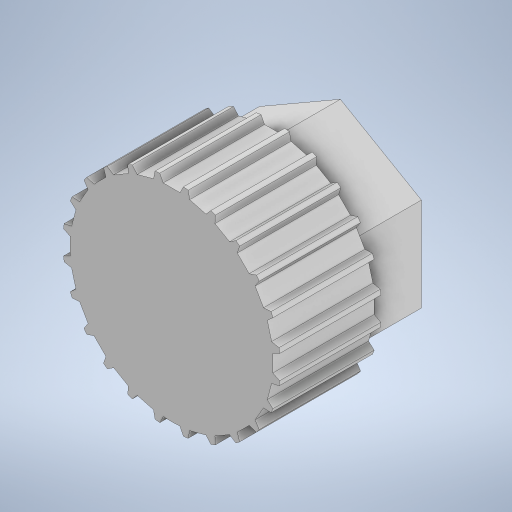
# Autodesk Inventor part: Nastavek Maillard Freewheel Tool
Saved by Autodesk Inventor 2023.3 (Build 273359000, 359)
## iProperties
Created: 2024-05-29
Part Number: Nastavek Maillard Freewheel Tool
Material: Generic
Document SubType Name: Modeling
Designer: David Zindović
Density: 1 g/cm^3
Appearance: Default
Author: David Zindović
Autodesk Inventor part; units mm, degrees
ref_plane "YZ Plane" through (0, 0, 0) normal (1, 0, 0) x (0, 1, 0)
ref_plane "XZ Plane" through (0, 0, 0) normal (0, 1, 0) x (-1, 0, 0)
ref_plane "XY Plane" through (0, 0, 0) normal (0, 0, 1) x (1, 0, 0)
sketch "Sketch1" plane through (0, 0, 0) normal (0, 0, 1) x (1, 0, 0)
  circle A0 centre (0, 0) radius 17.25
  circle A1 centre (0, 0) radius 16.1
  circle A2 centre (0, 0) radius 15
  line L0 (-1.25, -15.0046) -> (1.25, -15.0046)
  line L1 (-1.75, -16.0046) -> (1.75, -16.0046)
  line L2 (1.75, -16.0046) -> (1.25, -15.0046)
  line L3 (-1.75, -16.0046) -> (-1.25, -15.0046)
  line L4 (-1.25, -15.0046) -> (-1.2227, -14.9501)
  line L5 (1.25, -15.0046) -> (1.2227, -14.9501)
  line L6 (2.6761, -14.8169) -> (5.0909, -14.1698)
  line L7 (2.4519, -15.9122) -> (2.6761, -14.8169)
  line L8 (2.6761, -14.8169) -> (2.6883, -14.7571)
  line L9 (5.8327, -15.0063) -> (5.0909, -14.1698)
  line L10 (5.0909, -14.1698) -> (5.0504, -14.1242)
  line L11 (6.4198, -13.6194) -> (8.5848, -12.3694)
  line L12 (6.4868, -14.7354) -> (6.4198, -13.6194)
  line L13 (6.4198, -13.6194) -> (6.4161, -13.5585)
  line L14 (9.5178, -12.9854) -> (8.5848, -12.3694)
  line L15 (8.5848, -12.3694) -> (8.534, -12.3358)
  line L16 (9.726, -11.4937) -> (11.4937, -9.726)
  line L17 (10.0795, -12.5544) -> (9.726, -11.4937)
  line L18 (9.726, -11.4937) -> (9.7067, -11.4359)
  line L19 (12.5544, -10.0795) -> (11.4937, -9.726)
  line L20 (11.4937, -9.726) -> (11.4359, -9.7067)
  line L21 (12.3694, -8.5848) -> (13.6194, -6.4198)
  line L22 (12.9854, -9.5178) -> (12.3694, -8.5848)
  line L23 (12.3694, -8.5848) -> (12.3358, -8.534)
  line L24 (14.7354, -6.4868) -> (13.6194, -6.4198)
  line L25 (13.6194, -6.4198) -> (13.5585, -6.4161)
  line L26 (14.1698, -5.0909) -> (14.8169, -2.6761)
  line L27 (15.0063, -5.8327) -> (14.1698, -5.0909)
  line L28 (14.1698, -5.0909) -> (14.1242, -5.0504)
  line L29 (15.9122, -2.4519) -> (14.8169, -2.6761)
  line L30 (14.8169, -2.6761) -> (14.7571, -2.6883)
  line L31 (15.0046, -1.25) -> (15.0046, 1.25)
  line L32 (16.0046, -1.75) -> (15.0046, -1.25)
  line L33 (15.0046, -1.25) -> (14.9501, -1.2227)
  line L34 (16.0046, 1.75) -> (15.0046, 1.25)
  line L35 (15.0046, 1.25) -> (14.9501, 1.2227)
  line L36 (14.8169, 2.6761) -> (14.1698, 5.0909)
  line L37 (15.9122, 2.4519) -> (14.8169, 2.6761)
  line L38 (14.8169, 2.6761) -> (14.7571, 2.6883)
  line L39 (15.0063, 5.8327) -> (14.1698, 5.0909)
  line L40 (14.1698, 5.0909) -> (14.1242, 5.0504)
  line L41 (13.6194, 6.4198) -> (12.3694, 8.5848)
  line L42 (14.7354, 6.4868) -> (13.6194, 6.4198)
  line L43 (13.6194, 6.4198) -> (13.5585, 6.4161)
  line L44 (12.9854, 9.5178) -> (12.3694, 8.5848)
  line L45 (12.3694, 8.5848) -> (12.3358, 8.534)
  line L46 (11.4937, 9.726) -> (9.726, 11.4937)
  line L47 (12.5544, 10.0795) -> (11.4937, 9.726)
  line L48 (11.4937, 9.726) -> (11.4359, 9.7067)
  line L49 (10.0795, 12.5544) -> (9.726, 11.4937)
  line L50 (9.726, 11.4937) -> (9.7067, 11.4359)
  line L51 (8.5848, 12.3694) -> (6.4198, 13.6194)
  line L52 (9.5178, 12.9854) -> (8.5848, 12.3694)
  line L53 (8.5848, 12.3694) -> (8.534, 12.3358)
  line L54 (6.4868, 14.7354) -> (6.4198, 13.6194)
  line L55 (6.4198, 13.6194) -> (6.4161, 13.5585)
  line L56 (5.0909, 14.1698) -> (2.6761, 14.8169)
  line L57 (5.8327, 15.0063) -> (5.0909, 14.1698)
  line L58 (5.0909, 14.1698) -> (5.0504, 14.1242)
  line L59 (2.4519, 15.9122) -> (2.6761, 14.8169)
  line L60 (2.6761, 14.8169) -> (2.6883, 14.7571)
  line L61 (1.25, 15.0046) -> (-1.25, 15.0046)
  line L62 (1.75, 16.0046) -> (1.25, 15.0046)
  line L63 (1.25, 15.0046) -> (1.2227, 14.9501)
  line L64 (-1.75, 16.0046) -> (-1.25, 15.0046)
  line L65 (-1.25, 15.0046) -> (-1.2227, 14.9501)
  line L66 (-2.6761, 14.8169) -> (-5.0909, 14.1698)
  line L67 (-2.4519, 15.9122) -> (-2.6761, 14.8169)
  line L68 (-2.6761, 14.8169) -> (-2.6883, 14.7571)
  line L69 (-5.8327, 15.0063) -> (-5.0909, 14.1698)
  line L70 (-5.0909, 14.1698) -> (-5.0504, 14.1242)
  line L71 (-6.4198, 13.6194) -> (-8.5848, 12.3694)
  line L72 (-6.4868, 14.7354) -> (-6.4198, 13.6194)
  line L73 (-6.4198, 13.6194) -> (-6.4161, 13.5585)
  line L74 (-9.5178, 12.9854) -> (-8.5848, 12.3694)
  line L75 (-8.5848, 12.3694) -> (-8.534, 12.3358)
  line L76 (-9.726, 11.4937) -> (-11.4937, 9.726)
  line L77 (-10.0795, 12.5544) -> (-9.726, 11.4937)
  line L78 (-9.726, 11.4937) -> (-9.7067, 11.4359)
  line L79 (-12.5544, 10.0795) -> (-11.4937, 9.726)
  line L80 (-11.4937, 9.726) -> (-11.4359, 9.7067)
  line L81 (-12.3694, 8.5848) -> (-13.6194, 6.4198)
  line L82 (-12.9854, 9.5178) -> (-12.3694, 8.5848)
  line L83 (-12.3694, 8.5848) -> (-12.3358, 8.534)
  line L84 (-14.7354, 6.4868) -> (-13.6194, 6.4198)
  line L85 (-13.6194, 6.4198) -> (-13.5585, 6.4161)
  line L86 (-14.1698, 5.0909) -> (-14.8169, 2.6761)
  line L87 (-15.0063, 5.8327) -> (-14.1698, 5.0909)
  line L88 (-14.1698, 5.0909) -> (-14.1242, 5.0504)
  line L89 (-15.9122, 2.4519) -> (-14.8169, 2.6761)
  line L90 (-14.8169, 2.6761) -> (-14.7571, 2.6883)
  line L91 (-15.0046, 1.25) -> (-15.0046, -1.25)
  line L92 (-16.0046, 1.75) -> (-15.0046, 1.25)
  line L93 (-15.0046, 1.25) -> (-14.9501, 1.2227)
  line L94 (-16.0046, -1.75) -> (-15.0046, -1.25)
  line L95 (-15.0046, -1.25) -> (-14.9501, -1.2227)
  line L96 (-14.8169, -2.6761) -> (-14.1698, -5.0909)
  line L97 (-15.9122, -2.4519) -> (-14.8169, -2.6761)
  line L98 (-14.8169, -2.6761) -> (-14.7571, -2.6883)
  line L99 (-15.0063, -5.8327) -> (-14.1698, -5.0909)
  line L100 (-14.1698, -5.0909) -> (-14.1242, -5.0504)
  line L101 (-13.6194, -6.4198) -> (-12.3694, -8.5848)
  line L102 (-14.7354, -6.4868) -> (-13.6194, -6.4198)
  line L103 (-13.6194, -6.4198) -> (-13.5585, -6.4161)
  line L104 (-12.9854, -9.5178) -> (-12.3694, -8.5848)
  line L105 (-12.3694, -8.5848) -> (-12.3358, -8.534)
  line L106 (-11.4937, -9.726) -> (-9.726, -11.4937)
  line L107 (-12.5544, -10.0795) -> (-11.4937, -9.726)
  line L108 (-11.4937, -9.726) -> (-11.4359, -9.7067)
  line L109 (-10.0795, -12.5544) -> (-9.726, -11.4937)
  line L110 (-9.726, -11.4937) -> (-9.7067, -11.4359)
  line L111 (-8.5848, -12.3694) -> (-6.4198, -13.6194)
  line L112 (-9.5178, -12.9854) -> (-8.5848, -12.3694)
  line L113 (-8.5848, -12.3694) -> (-8.534, -12.3358)
  line L114 (-6.4868, -14.7354) -> (-6.4198, -13.6194)
  line L115 (-6.4198, -13.6194) -> (-6.4161, -13.5585)
  line L116 (-5.0909, -14.1698) -> (-2.6761, -14.8169)
  line L117 (-5.8327, -15.0063) -> (-5.0909, -14.1698)
  line L118 (-5.0909, -14.1698) -> (-5.0504, -14.1242)
  line L119 (-2.4519, -15.9122) -> (-2.6761, -14.8169)
  line L120 (-2.6761, -14.8169) -> (-2.6883, -14.7571)
  point P0 (0, -16.0046)
  point P1 (0, -15.0046)
  point P2 (1.75, -16.0046)
  point P3 (3.8835, -14.4933)
  point P4 (7.5023, -12.9944)
  point P5 (10.6099, -10.6099)
  point P6 (12.9944, -7.5023)
  point P7 (14.4933, -3.8835)
  point P8 (15.0046, 0)
  point P9 (14.4933, 3.8835)
  point P10 (12.9944, 7.5023)
  point P11 (10.6099, 10.6099)
  point P12 (7.5023, 12.9944)
  point P13 (3.8835, 14.4933)
  point P14 (0, 15.0046)
  point P15 (-3.8835, 14.4933)
  point P16 (-7.5023, 12.9944)
  point P17 (-10.6099, 10.6099)
  point P18 (-12.9944, 7.5023)
  point P19 (-14.4933, 3.8835)
  point P20 (-15.0046, 0)
  point P21 (-14.4933, -3.8835)
  point P22 (-12.9944, -7.5023)
  point P23 (-10.6099, -10.6099)
  point P24 (-7.5023, -12.9944)
  point P25 (-3.8835, -14.4933)
  dimension "d1" = 32.2
  dimension "d0" = 34.5
  dimension "d2" = 30
  dimension "d3" = 2.5
  dimension "d4" = 3.5
  dimension "d5" = 1
  dimension "d20" = 360
  constraints: 242 end point, 3 coincident, 2 centre point, 2 collinear, 2 horizontal, 2 midpoint, 2 point on circle, 2 vertical alignment, 292 other
  measures "d0" diameter of A0
  measures "d2" diameter of A2
  measures "d3" distance of L0.start L0.end
  measures "d4" distance of L1.start L1.end
  measures "d5" distance between parallel lines of L0 L1
extrude "Extrusion1" add sketch "Sketch1" along normal blind 15 contours L34 L35 A2 L38 L37 A1 | A1 L29 L30 A2 L33 L32 | L31 L33 A2 L35 | L39 L40 A2 L43 L42 A1 | L38 A2 L40 L36 | A2 | A1 L24 L25 A2 L28 L27 | L26 L28 A2 L30 | L44 L45 A2 L48 L47 A1 | L43 A2 L45 L41 | A1 L19 L20 A2 L23 L22 | L21 L23 A2 L25 | L49 L50 A2 L53 L52 A1 | L48 A2 L50 L46 | A1 L14 L15 A2 L18 L17 | L16 L18 A2 L20 | L54 L55 A2 L58 L57 A1 | L53 A2 L55 L51 | A1 L9 L10 A2 L13 L12 | L11 L13 A2 L15 | L59 L60 A2 L63 L62 A1 | L58 A2 L60 L56 | A1 L2 L5 A2 L8 L7 | L6 L8 A2 L10 | L64 L65 A2 L68 L67 A1 | L63 A2 L65 L61 | A1 L119 L120 A2 L4 L3 | L69 L70 A2 L73 L72 A1 | L68 A2 L70 L66 | A1 L114 L115 A2 L118 L117 | L116 L118 A2 L120 | L74 L75 A2 L78 L77 A1 | L73 A2 L75 L71 | A1 L109 L110 A2 L113 L112 | L111 L113 A2 L115 | L79 L80 A2 L83 L82 A1 | L78 A2 L80 L76 | A1 L104 L105 A2 L108 L107 | L106 L108 A2 L110 | L84 L85 A2 L88 L87 A1 | L83 A2 L85 L81 | A1 L99 L100 A2 L103 L102 | L101 L103 A2 L105 | L89 L90 A2 L93 L92 A1 | L88 A2 L90 L86 | A1 L94 L95 A2 L98 L97 | L96 L98 A2 L100 | L93 A2 L95 L91
sketch "Sketch2" plane through (0, 0, 0) normal (0, 0, -1) x (-1, 0, 0)
  line L0 (12, 6.9282) -> (12, -6.9282)
  line L1 (12, -6.9282) -> (0, -13.8564)
  line L2 (0, -13.8564) -> (-12, -6.9282)
  line L3 (-12, -6.9282) -> (-12, 6.9282)
  line L4 (-12, 6.9282) -> (0, 13.8564)
  line L5 (0, 13.8564) -> (12, 6.9282)
  point P0 (0, 0)
  point P1 (0, 0)
  dimension "d12" = 24
  constraints: 12 end point, 1 coincident, 1 vertical alignment, 13 other
  measures "d12" distance between parallel lines of L3 L0
extrude "Extrusion2" add sketch "Sketch2" along normal blind 10
sketch "Sketch3" plane through (0, 0, -10) normal (0, 0, -1) x (-1, 0, 0)
  circle A0 centre (0, 0) radius 7.5
  dimension "d15" = 15
  constraints: 1 centre point, 1 coincident
  measures "d15" diameter of A0
extrude "Extrusion3" [suppressed]
sketch "Sketch4" plane through (0, 0, 0) normal (1, 0, 0) x (0, 1, 0)
  line L0 (20.8545, -11.8216) -> (-20.3089, -11.8216)
  line L1 (-20.3089, -11.8216) -> (-20.3089, 5.7592)
  line L2 (-20.3089, 5.7592) -> (20.8545, 5.7592)
  line L3 (20.8545, 5.7592) -> (20.8545, -11.8216)
  point P0 (0, 0)
  constraints: 8 end point, 2 parallel, 1 horizontal, 1 perpendicular
extrude "Extrusion4" [suppressed]
body "Solid1"
